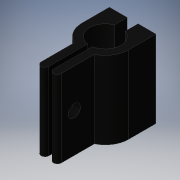
# Autodesk Inventor part: pen holder 3
Saved by Autodesk Inventor 2016 (Build 200138000, 138)
## iProperties
Created: 2017-03-27
Part Number: pen holder 3
Material: PBT Plastic
Document SubType Name: Modeling
Designer: jwillauer
Density: 1.31 g/cm^3
Appearance: Glossy - Black
Author: jwillauer
Autodesk Inventor part; units mm, degrees
ref_plane "YZ Plane" through (0, 0, 0) normal (1, 0, 0) x (0, 1, 0)
ref_plane "XZ Plane" through (0, 0, 0) normal (0, 1, 0) x (-1, 0, 0)
ref_plane "XY Plane" through (0, 0, 0) normal (0, 0, 1) x (1, 0, 0)
sketch "Sketch1" plane through (0, 0, 0) normal (0, 1, 0) x (-1, 0, 0)
  line L0 (-0.762, 12.7) -> (-0.762, 17.7225)
  line L1 (0.762, 12.7) -> (0.762, 17.7225)
  line L2 (-3.302, 12.7) -> (-3.302, 17.7225)
  line L3 (3.302, 12.7) -> (3.302, 17.7225)
  line L4 (3.302, 12.7) -> (3.302, 6.8674)
  line L5 (-3.302, 12.7) -> (-3.302, 6.8674)
  line L6 (-2.032, 18.9925) -> (-2.032, 18.9925)
  line L7 (2.032, 18.9925) -> (2.032, 18.9925)
  arc A0 (3.302, 17.7225) -> (2.032, 18.9925) centre (2.032, 17.7225) ccw
  arc A1 (2.032, 18.9925) -> (0.762, 17.7225) centre (2.032, 17.7225) ccw
  arc A2 (-0.762, 17.7225) -> (-2.032, 18.9925) centre (-2.032, 17.7225) ccw
  arc A3 (-2.032, 18.9925) -> (-3.302, 17.7225) centre (-2.032, 17.7225) ccw
  arc A4 (-0.762, 5.0225) -> (0.762, 5.0225) centre (0, 0) ccw
  line L8 (0.762, 12.7) -> (0.762, 5.0225)
  line L9 (-0.762, 12.7) -> (-0.762, 5.0225)
  arc A5 (-3.302, 6.8674) -> (-7.6187, -0.1405) centre (0, 0) ccw
  arc A6 (7.6187, -0.1405) -> (3.302, 6.8674) centre (0, 0) ccw
  line L10 (7.6187, -8.9561) -> (-7.6187, -8.9561)
  line L11 (7.6187, -8.9561) -> (7.6187, 0.1405)
  line L12 (-7.6187, -8.9561) -> (-7.6187, 0.1405)
  dimension "d3" = 2.54
  dimension "d4" = 2.54
  dimension "d5" = 1.27
  dimension "d6" = 10.16
  dimension "d7" = 1.524
  dimension "d8" = 1.524
  dimension "d9" = 12.7
  dimension "d10" = 12.7
  constraints: 26 end point, 16 point on circle, 8 tangent, 7 centre point, 4 equal length, 3 equal radius, 2 coincident, 2 point on line, 1 horizontal, 1 perpendicular, 1 vertical
  measures "d3" distance between parallel lines of L0 L2
  measures "d4" distance between parallel lines of L1 L3
  measures "d5" radius of A0
  measures "d6" diameter of A4
  measures "d7" distance between parallel lines of L0 L1
  measures "d8" distance between parallel lines of L9 L8
  measures "d9" vertical distance of L9.end A2.centre
  measures "d10" vertical distance of L8.end A0.centre
extrude "Extrusion1" add sketch "Sketch1" along normal blind 25.4
sketch "Sketch3" plane through (3.302, 0, 17.7225) normal (1, 0, 0) x (0, 0, -1)
  line L0 (0, 25.4) -> (10.8551, 25.4) projected
  point P0 (17.7225, 0)
  point P1 (4.2489, 12.7)
  dimension "d24" = 12.7
  measures "d24" distance from line of L0 point (4.249, 12.7)
hole "Hole2" at (3.302, 12.7, 13.4736) direction (-1, 0, 0) diameter 4.064 end through all
sketch "Sketch5" plane through (7.6187, 0, -8.9561) normal (0, 0, -1) x (-1, 0, 0)
  line L0 (2.5387, 0) -> (12.6987, 0) projected
  point P0 (7.6187, 0)
  point P1 (7.6187, 12.7)
  point P2 (8.3807, 0)
  point P3 (6.8567, 0)
  dimension "d34" = 12.7
  measures "d34" distance from line of L0 point (7.619, 12.7)
hole "Hole3" at (0, 12.7, -8.9561) direction (0, 0, 1) diameter 3.556 depth 4.7625 tip angle 118
chamfer "Chamfer2" distance 2.286 angle 45 1 edges at (-0.0006, 10.922, -5.08)
sketch "Sketch6" plane through (7.6187, 0, -8.9561) normal (0, 0, -1) x (-1, 0, 0)
  circle A0 centre (7.6187, 12.7) radius 1.778 projected
  line L0 (5.8407, 12.7) -> (9.3967, 12.7)
  line L1 (9.3967, 12.7) -> (9.3967, 25.4084)
  line L2 (9.3967, 25.4084) -> (5.8407, 25.4084)
  line L3 (5.8407, 25.4084) -> (5.8407, 12.7)
  point P0 (7.6187, 0)
  constraints: 8 end point, 2 parallel, 1 horizontal, 1 horizontal alignment, 1 perpendicular, 1 other
extrude "Extrusion2" cut sketch "Sketch6" against normal blind 6.35 contours L0 A0 | A0 L3 L2 L1 picked at (8.0623, 13.093)
equation "\"d10\" = d9"
body "Solid1"
